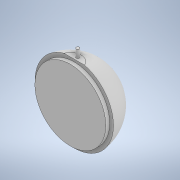
# Autodesk Inventor part: bulb turning point
Saved by Autodesk Inventor 2022 (Build 260153000, 153)
## iProperties
Created: 2022-03-14
Part Number: bulb turning point
Material: Generic
Document SubType Name: Modeling
Designer: mogje
Density: 1 g/cm^3
Appearance: Default
Author: mogje
Autodesk Inventor part; units mm, degrees
ref_plane "YZ Plane" through (0, 0, 0) normal (1, 0, 0) x (0, 1, 0)
ref_plane "XZ Plane" through (0, 0, 0) normal (0, 1, 0) x (-1, 0, 0)
ref_plane "XY Plane" through (0, 0, 0) normal (0, 0, 1) x (1, 0, 0)
sketch "Sketch6" plane through (0, 0, 0) normal (0, 0, 1) x (1, 0, 0)
  arc A0 (-31.75, 0) -> (31.75, 0) centre (0, 0) ccw
  line L0 (-31.75, 0) -> (31.75, 0)
  constraints: 2 end point, 2 point on circle, 1 centre point, 1 coincident, 1 horizontal
revolve "Revolution2" add sketch "Sketch6" angle 180 about axis through (-31.75, 0, 0) along (1, 0, 0)
sketch "Sketch9" plane through (0, 0, 0) normal (0, 0, 1) x (1, 0, 0)
  circle A0 centre (0, 0) radius 31.75
  constraints: 1 centre point, 1 coincident
extrude "Extrusion5" cut sketch "Sketch9" against normal blind 3.175
sketch "Sketch10" plane through (0, 0, -3.175) normal (0, 0, 1) x (1, 0, 0)
  circle A0 centre (0, 0) radius 28.575
  constraints: 1 centre point, 1 coincident
extrude "Extrusion6" add sketch "Sketch10" along normal blind 3.175
sketch "Sketch11" plane through (0, 0, 0) normal (0, 1, 0) x (-1, 0, 0)
  arc A0 (-31.7973, 0) -> (31.7973, 0) centre (0, 0) ccw
  line L0 (31.7973, 0) -> (-31.7973, 0)
  line L1 (-31.5909, -3.175) -> (31.5909, -3.175) projected
  constraints: 2 end point, 2 point on circle, 1 centre point, 1 coincident, 1 parallel
extrude "Extrusion7" cut sketch "Sketch11" along normal blind 30.48 and the other way blind 31.75 keep common part
sketch "Sketch12" plane through (0, 30.48, 0) normal (0, 1, 0) x (1, 0, 0)
  line L0 (28.575, 3.175) -> (-28.575, 3.175) projected
  line L1 (0, 3.175) -> (0, 8.89)
  arc A0 (8.3037, 3.175) -> (-8.3037, 3.175) centre (0, 0) ccw projected
  line L2 (0, 3.175) -> (0, 6.0325)
  circle A1 centre (0, 6.0325) radius 1.27
  dimension "d29" = 5.715
  dimension "d30" = 2.8575
  dimension "d31" = 2.54
  constraints: 4 end point, 2 midpoint, 1 centre point, 1 coincident, 1 point on circle, 1 vertical
  measures "d29" distance of L1.start L1.end
  measures "d30" distance of L1.start L2.end
  measures "d31" diameter of A1
extrude "Extrusion8" add sketch "Sketch12" along normal blind 6.35 contours A1 L1 | L1 A1
body "Solid2"
